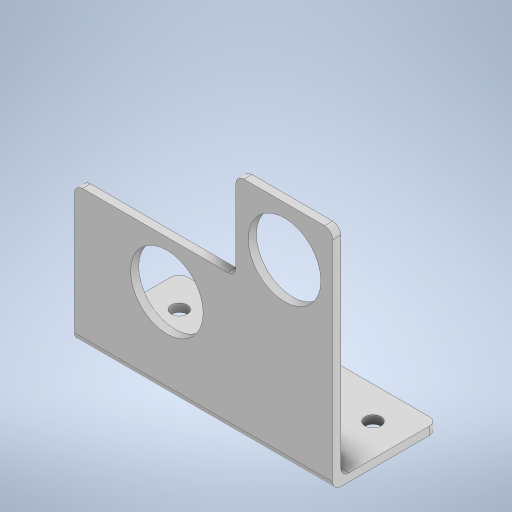
# Autodesk Inventor part: 4-bar intake mount(alt)
Saved by Autodesk Inventor 2023 (Build 270158030, 158C)
## iProperties
Created: 2022-07-18
Part Number: 4-bar intake mount(alt)
Material: Generic
Document SubType Name: Modeling
Designer: kt1040502
Density: 1 g/cm^3
Appearance: Default
Author: kt1040502
Autodesk Inventor part; units mm, degrees
ref_plane "YZ Plane" through (0, 0, 0) normal (1, 0, 0) x (0, 1, 0)
ref_plane "XZ Plane" through (0, 0, 0) normal (0, 1, 0) x (-1, 0, 0)
ref_plane "XY Plane" through (0, 0, 0) normal (0, 0, 1) x (1, 0, 0)
sketch "Sketch1" plane through (0, 0, 0) normal (0, 0, 1) x (1, 0, 0)
  line L0 (762, 0) -> (762, -101.6)
  line L1 (762, -101.6) -> (0, -101.6)
  line L2 (0, -101.6) -> (0, 0)
  line L3 (194.457, 486.6085) -> (233.372, 453.9549)
  line L4 (233.372, 453.9549) -> (102.7576, 298.2946)
  line L5 (102.7576, 298.2946) -> (63.8425, 330.9483)
  line L6 (63.8425, 330.9483) -> (194.457, 486.6085)
  line L7 (-316.8542, 110.7002) -> (-152.9915, 230.8635)
  line L8 (-152.9915, 230.8635) -> (-122.9506, 189.8979)
  line L9 (-122.9506, 189.8979) -> (-286.8134, 69.7345)
  line L10 (-286.8134, 69.7345) -> (-316.8542, 110.7002)
  circle A0 centre (97.7035, 16.2291) radius 358.4366 construction
  line L11 (-240.3853, 135.2786) -> (97.7035, 16.2291) construction
  line L12 (97.7035, 16.2291) -> (132.2805, 372.994) construction
  circle A1 centre (144.0057, 50.3583) radius 362.156 construction
  line L13 (144.0057, 50.3583) -> (164.9341, 411.9091) construction
  line L14 (144.0057, 50.3583) -> (-199.4196, 165.3194) construction
  circle A2 centre (-240.3853, 135.2786) radius 12.7
  circle A3 centre (-199.4196, 165.3194) radius 12.7
  circle A4 centre (132.2805, 372.994) radius 12.7
  circle A5 centre (164.9341, 411.9091) radius 12.7
  circle A6 centre (97.7035, 16.2291) radius 12.7
  circle A7 centre (144.0057, 50.3583) radius 12.7
  line L15 (-199.4196, 165.3194) -> (144.0057, 50.3583) construction
  arc A8 (-215.4061, 202.6622) -> (-230.8062, 191.1057) centre (-199.4196, 165.3194) ccw
  arc A9 (131.5057, 48.1134) -> (132.3942, 55.5025) centre (144.0057, 50.3583) ccw
  line L16 (-240.3853, 135.2786) -> (97.7035, 16.2291) construction
  line L17 (-244.6034, 123.2995) -> (93.4854, 4.2501)
  line L18 (101.9216, 28.2081) -> (-236.1671, 147.2576)
  arc A10 (-236.1671, 147.2576) -> (-244.6034, 123.2995) centre (-240.3853, 135.2786) ccw
  arc A11 (93.4854, 4.2501) -> (101.9216, 28.2081) centre (97.7035, 16.2291) ccw
  line L19 (164.9341, 411.9091) -> (144.0057, 50.3583) construction
  line L20 (152.2553, 412.643) -> (131.3269, 51.0922)
  line L21 (156.6845, 49.6244) -> (177.6129, 411.1752)
  arc A12 (177.6129, 411.1752) -> (152.2553, 412.643) centre (164.9341, 411.9091) ccw
  arc A13 (131.3269, 51.0922) -> (156.6845, 49.6244) centre (144.0057, 50.3583) ccw
  line L22 (132.2805, 372.994) -> (97.7035, 16.2291) construction
  line L23 (119.6397, 374.2192) -> (85.0627, 17.4542)
  line L24 (110.3443, 15.004) -> (144.9213, 371.7689)
  arc A14 (144.9213, 371.7689) -> (119.6397, 374.2192) centre (132.2805, 372.994) ccw
  arc A15 (85.0627, 17.4542) -> (110.3443, 15.004) centre (97.7035, 16.2291) ccw
  line L25 (144.0057, 50.3583) -> (-199.4196, 165.3194) construction
  line L26 (148.0371, 62.4015) -> (-195.3881, 177.3626)
  line L27 (-203.451, 153.2763) -> (139.9743, 38.3151)
  arc A16 (139.9743, 38.3151) -> (148.0371, 62.4015) centre (144.0057, 50.3583) ccw
  arc A17 (-195.3881, 177.3626) -> (-203.451, 153.2763) centre (-199.4196, 165.3194) ccw
  line L28 (162.9213, 0) -> (162.9213, 31.75)
  line L29 (61.3213, 28.575) -> (61.3213, 0)
  line L30 (162.9213, 31.75) -> (124.8213, 31.75)
  line L31 (124.8213, 38.1) -> (124.8213, 66.675)
  line L32 (127.9963, 69.85) -> (159.7463, 69.85)
  line L33 (162.9213, 66.675) -> (162.9213, 31.75)
  arc A18 (162.9213, 66.675) -> (159.7463, 69.85) centre (159.7463, 66.675) ccw
  arc A19 (127.9963, 69.85) -> (124.8213, 66.675) centre (127.9963, 66.675) ccw
  circle A20 centre (144.0057, 50.3583) radius 14.2875
  circle A21 centre (97.7035, 16.2291) radius 14.2875
  line L34 (61.3213, 0) -> (61.3213, -6.35)
  line L35 (61.3213, -6.35) -> (162.9213, -6.35)
  line L36 (162.9213, -6.35) -> (162.9213, 0)
  line L37 (124.8213, 34.925) -> (121.541, 34.925)
  line L38 (121.6463, 34.925) -> (64.4963, 34.925)
  line L39 (61.3213, 31.75) -> (61.3213, 28.575)
  arc A22 (64.4963, 34.925) -> (61.3213, 31.75) centre (64.4963, 31.75) ccw
  arc A23 (121.6463, 34.925) -> (124.8213, 38.1) centre (121.6463, 38.1) ccw
  line L40 (61.3213, -6.35) -> (61.3213, -19.05)
  line L41 (61.3213, -19.05) -> (162.9213, -19.05)
  line L42 (162.9213, -19.05) -> (162.9213, -6.35)
  line L43 (61.3213, -15.875) -> (162.9213, -15.875)
  point P0 (213.9145, 470.2817)
  point P1 (83.3001, 314.6214)
  point P2 (-301.8338, 90.2173)
  point P3 (-27.7069, 107.8389)
  point P4 (-71.3409, 75.7538)
  point P5 (154.4699, 231.1337)
  point P6 (114.992, 194.6116)
  point P7 (-27.7069, 107.8389)
  point P8 (124.8213, 69.85)
  point P9 (162.9213, 69.85)
  point P10 (132.4127, 69.85)
  point P11 (132.2867, 67.6739)
  point P12 (141.8302, 64.4792)
  point P13 (131.7052, 57.6267)
  point P14 (126.6629, 69.5564)
  point P15 (61.3213, 34.925)
  point P16 (124.8213, 43.3876)
  point P17 (157.8552, 69.85)
  point P18 (157.0627, 56.1589)
  point P19 (133.7674, 40.3929)
  point P20 (86.6269, 33.5938)
  point P21 (82.8464, 34.925)
  point P22 (86.756, 34.925)
  dimension "d0" = 762
  dimension "d1" = 101.6
  dimension "d2" = 50.8
  dimension "d3" = 203.2
  dimension "d6" = 203.2
  dimension "d7" = 50.8
  dimension "d12" = 25.4
  dimension "d13" = 25.4
  dimension "d14" = 25.4
  dimension "d15" = 25.4
  dimension "d16" = 25.4
  dimension "d17" = 25.4
  dimension "d18" = 25.4
  dimension "d19" = 25.4
  dimension "d20" = 76.2
  dimension "d21" = 76.2
  dimension "d22" = 76.2
  dimension "d23" = 76.2
  dimension "d24" = 25.4
  dimension "d25" = 25.4
  dimension "d26" = 25.4
  dimension "d27" = 25.4
  dimension "d28" = 25.4
  dimension "d29" = 25.4
  dimension "d30" = 25.4
  dimension "d32" = 31.75
  dimension "d33" = 38.1
  dimension "d34" = 38.1
  dimension "d35" = 3.175
  dimension "d43" = 28.575
  dimension "d44" = 28.575
  dimension "d45" = 6.35
  dimension "d47" = 3.175
  dimension "d65" = 12.7
  dimension "d66" = 3.175
  constraints: 98 end point, 32 point on circle, 24 centre point, 24 tangent, 12 point on line, 11 perpendicular, 10 coincident, 10 parallel, 8 midpoint, 6 equal radius, 5 collinear, 2 vertical, 1 horizontal
  measures "d0" distance of L0.end L1.end
  measures "d1" distance of L0.start L0.end
  measures "d2" distance of L4.end L5.end
  measures "d3" distance of L3.end L4.end
  measures "d6" distance of L8.end L9.end
  measures "d7" distance of L7.end L8.end
  measures "d12" distance from line of L4 L12.end
  measures "d13" distance from line of L4 L13.end
  measures "d14" diameter of A2
  measures "d15" diameter of A3
  measures "d16" diameter of A4
  measures "d17" diameter of A5
  measures "d18" distance from line of L9 A2.centre
  measures "d19" distance from line of L9 L14.end
  measures "d20" distance from line of L3 L13.end
  measures "d21" distance from line of L5 L12.end
  measures "d22" distance from line of L10 L11.start
  measures "d23" distance from line of L8 L14.end
  measures "d24" diameter of A6
  measures "d25" diameter of A7
  measures "d26" diameter of A9
  measures "d27" diameter of A11
  measures "d28" diameter of A13
  measures "d29" diameter of A15
  measures "d30" diameter of A17
  measures "d32" distance of L28.end L28.start
  measures "d33" distance of point (124.821, 69.85) point (162.921, 69.85)
  measures "d34" distance of L30.end point (124.821, 69.85)
  measures "d35" radius of A18
  measures "d43" diameter of A20
  measures "d44" diameter of A21
  measures "d45" distance of L29.end L34.end
  measures "d47" radius of A22
  measures "d65" distance of L34.end L40.end
  measures "d66" distance between parallel lines of L41 L43
extrude "Extrusion1" add sketch "Sketch1" along normal blind 3.175 contours L32 A18 L33 L28 L36 L35 L34 L29 L17 A21 L24 L38 L37 A23 L31 L27 A20 L21 | L21 A20 L26 L20 L32 | L20 L26 A19 L32 | L26 A20 L20 | L20 A20 L27 L31 A19 L26 | L38 L24 A21 L18 L23 | L23 L18 L38 | L23 A21 L17 L29 L39 A22 L38 L18 | L18 A21 L23 | L42 L43 L40 L35 | L42 L41 L40 L43
sketch "Sketch7" plane through (0, 0, 0) normal (0, 0, -1) x (-1, 0, 0)
  line L0 (-162.9213, -19.05) -> (-162.9213, 66.675) projected
  line L1 (-61.3213, -19.05) -> (-162.9213, -19.05) projected
  line L2 (-61.3213, 31.75) -> (-61.3213, -19.05) projected
  line L3 (-162.9213, -15.875) -> (-61.3213, -15.875)
  point P0 (0, 0)
  dimension "d82" = 3.175
  constraints: 2 end point, 2 point on line, 1 perpendicular
  measures "d82" distance between parallel lines of L1 L3
extrude "Extrusion7" add sketch "Sketch7" along normal blind 38.1
fillet "Fillet3" radius 3.175 4 edges at (61.3213, -17.4625, -38.1) (162.9213, -17.4625, -38.1) (112.1213, -15.875, 0) (112.1213, -19.05, 3.175)
sketch "Sketch8" plane through (61.3213, -15.875, -3.175) normal (0, 1, 0) x (1, 0, 0)
  line L0 (101.6, 0) -> (101.6, 31.75) projected
  arc A0 (101.6, 31.75) -> (98.425, 34.925) centre (98.425, 31.75) ccw projected
  line L1 (3.175, 34.925) -> (98.425, 34.925) projected
  line L2 (0, 0) -> (0, 31.75) projected
  arc A1 (3.175, 34.925) -> (0, 31.75) centre (3.175, 31.75) ccw projected
  line L3 (101.6, 22.225) -> (0, 22.225)
  line L4 (0, 31.75) -> (0, -3.175) projected
  circle A2 centre (88.9, 22.225) radius 3.175
  circle A3 centre (63.5, 22.225) radius 3.175
  circle A4 centre (38.1, 22.225) radius 3.175
  circle A5 centre (12.7, 22.225) radius 3.175
  point P0 (-61.3213, -3.175)
  dimension "d86" = 12.7
  dimension "d87" = 6.35
  dimension "d88" = 6.35
  dimension "d89" = 6.35
  dimension "d90" = 6.35
  dimension "d91" = 12.7
  dimension "d92" = 25.4
  dimension "d93" = 25.4
  dimension "d94" = 25.4
  constraints: 6 point on line, 4 centre point, 2 end point, 1 perpendicular
  measures "d86" distance between parallel lines of L1 L3
  measures "d87" diameter of A2
  measures "d88" diameter of A3
  measures "d89" diameter of A4
  measures "d90" diameter of A5
  measures "d91" distance from line of A2.centre L0
  measures "d92" distance of A3.centre A2.centre
  measures "d93" distance of A4.centre A3.centre
  measures "d94" distance of A5.centre A4.centre
extrude "Extrusion8" cut sketch "Sketch8" against normal blind 38.1 contours A2 L3 | L3 A2 | A3 L3 | L3 A3 | A4 L3 | L3 A4 | A5 L3 | L3 A5
body "Solid1"
